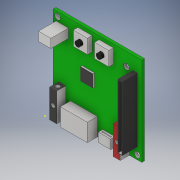
# Autodesk Inventor part: lab 04
Saved by Autodesk Inventor 2017 (Build 210142000, 142)
## iProperties
Created: 2016-10-26
Part Number: lab 04
Material: Generic
Document SubType Name: Modeling
Designer: radrajith
Density: 1 g/cm^3
Appearance: Default
Author: radrajith
Autodesk Inventor part; units mm, degrees
ref_plane "YZ Plane" through (0, 0, 0) normal (1, 0, 0) x (0, 1, 0)
ref_plane "XZ Plane" through (0, 0, 0) normal (0, 1, 0) x (-1, 0, 0)
ref_plane "XY Plane" through (0, 0, 0) normal (0, 0, 1) x (1, 0, 0)
sketch "Sketch1" plane through (0, 0, 0) normal (0, 0, 1) x (1, 0, 0)
  line L0 (0, 0) -> (50, 0)
  line L1 (50, 0) -> (50, 50)
  line L2 (50, 50) -> (0, 50)
  line L3 (0, 50) -> (0, 0)
  circle A0 centre (47.5, 2.5) radius 1.6
  circle A1 centre (41.39, 42.5) radius 1.6
  circle A2 centre (2.5, 47.5) radius 1.6
  dimension "d0" = 50
  dimension "d1" = 50
  dimension "d2" = 3.2
  dimension "d3" = 3.2
  dimension "d4" = 3.2
  constraints: 8 end point, 3 centre point, 2 parallel, 1 horizontal, 1 perpendicular
  measures "d0" distance of L2.end L1.end
  measures "d1" distance of L1.end L0.end
  measures "d2" diameter of A0
  measures "d3" diameter of A1
  measures "d4" diameter of A2
extrude "Extrusion1" add sketch "Sketch1" along normal blind 1.6
sketch "Sketch2" plane through (0, 0, 1.6) normal (0, 0, 1) x (1, 0, 0)
  line L0 (23.4, 30.52) -> (16.4, 30.52)
  line L1 (16.4, 30.52) -> (16.4, 23.52)
  line L2 (16.4, 23.52) -> (23.4, 23.52)
  line L3 (23.4, 23.52) -> (23.4, 30.52)
  point P0 (0, 0)
  dimension "d18" = 7
  dimension "d19" = 7
  constraints: 8 end point, 2 parallel, 1 horizontal, 1 perpendicular
  measures "d18" distance of L2.end L1.end
  measures "d19" distance of L1.end L0.end
extrude "Extrusion2" add sketch "Sketch2" along normal blind 1
sketch "Sketch3" plane through (0, 0, 1.6) normal (0, 0, 1) x (1, 0, 0)
  line L0 (47.541022, 6.34) -> (45.001022, 6.34)
  line L1 (45.001022, 6.34) -> (45.001022, 42.5)
  line L2 (45.001022, 42.5) -> (47.541022, 42.5)
  line L3 (47.541022, 42.5) -> (47.541022, 6.34)
  point P0 (0, 0)
  dimension "d11" = 2.54
  dimension "d12" = 36.16
  constraints: 8 end point, 2 parallel, 1 horizontal, 1 perpendicular
  measures "d11" distance of L1.end L2.end
  measures "d12" distance of L0.end L1.end
extrude "Extrusion3" add sketch "Sketch3" along normal blind 8.5
sketch "Sketch5" plane through (0, 0, 10.1) normal (0, 0, 1) x (1, 0, 0)
  line L0 (47.269103, 42.183511) -> (45.268765, 42.183511)
  line L1 (45.268765, 42.183511) -> (45.268765, 6.547483)
  line L2 (45.268765, 6.547483) -> (47.269103, 6.547483)
  line L3 (47.269103, 6.547483) -> (47.269103, 42.183511)
  point P0 (0, 0)
  constraints: 8 end point, 2 parallel, 1 horizontal, 1 perpendicular
extrude "Extrusion4" cut sketch "Sketch5" along normal mid plane 8
sketch "Sketch6" plane through (0, 0, 0) normal (0, -1, 0) x (1, 0, 0)
  line L0 (43, 1.6) -> (39, 1.6)
  line L1 (39, 1.6) -> (39, 6.75)
  line L2 (39, 6.75) -> (43, 6.75)
  line L3 (43, 6.75) -> (43, 1.6)
  line L4 (7.153325, 1.6) -> (3.153325, 1.6)
  line L5 (3.153325, 1.6) -> (3.153325, 6.75)
  line L6 (3.153325, 6.75) -> (7.153325, 6.75)
  line L7 (7.153325, 6.75) -> (7.153325, 1.6)
  line L8 (43, 1.6) -> (39, 1.6)
  line L9 (39, 1.6) -> (39, 6.75)
  line L10 (39, 6.75) -> (43, 6.75)
  line L11 (43, 6.75) -> (43, 1.6)
  point P0 (0, 0)
  dimension "d20" = 4
  dimension "d21" = 5.15
  dimension "d22" = 4
  dimension "d23" = 5.15
  dimension "d24" = 4
  dimension "d25" = 5.15
  constraints: 24 end point, 6 parallel, 3 horizontal, 3 perpendicular
  measures "d20" distance of L1.end L2.end
  measures "d21" distance of L0.end L1.end
  measures "d22" distance of L6.start L6.end
  measures "d23" distance of L5.start L6.start
  measures "d24" distance of L10.start L10.end
  measures "d25" distance of L9.start L10.start
extrude "Extrusion5" add sketch "Sketch6" against normal blind 16
hole "Hole1" at (41, 0, 4.175) direction (0, 1, 0) diameter 2.2 end through all
hole "Hole2" at (5.153325, 0, 4.175) direction (0, 1, 0) diameter 2.2 end through all
sketch "Sketch7" plane through (0, 0, 0) normal (0, -1, 0) x (1, 0, 0)
  line L0 (35, 4.100037) -> (28, 4.100037)
  line L1 (28, 4.100037) -> (28, 1.600037)
  line L2 (28, 1.600037) -> (35, 1.600037)
  line L3 (35, 1.600037) -> (35, 4.100037)
  point P0 (0, 0)
  dimension "d47" = 7
  dimension "d48" = 2.5
  constraints: 8 end point, 2 parallel, 1 horizontal, 1 perpendicular
  measures "d47" distance of L2.end L1.end
  measures "d48" distance of L1.end L0.end
extrude "Extrusion6" add sketch "Sketch7" against normal blind 5.1
shell "Shell1" thickness 1 removed faces 2 at (30.333333, 0, 3.266704) at (30.333333, 5.1, 3.266704)
sketch "Sketch8" plane through (0, 0, 0) normal (0, -1, 0) x (1, 0, 0)
  line L0 (25, 7.31808) -> (9.8, 7.31808)
  line L1 (9.8, 7.31808) -> (9.8, 1.59808)
  line L2 (9.8, 1.59808) -> (25, 1.59808)
  line L3 (25, 1.59808) -> (25, 7.31808)
  point P0 (0, 0)
  dimension "d52" = 15.2
  dimension "d56" = 5.72
  constraints: 8 end point, 2 parallel, 1 horizontal, 1 perpendicular
  measures "d52" distance of L2.end L1.end
  measures "d56" distance between parallel lines of L0 L2
extrude "Extrusion7" add sketch "Sketch8" against normal blind 10
sketch "Sketch10" plane through (0, 0, 0) normal (0, -1, 0) x (1, 0, 0)
  line L0 (11.3, 6.482537) -> (23.5, 6.482537)
  line L1 (23.5, 6.482537) -> (23.5, 2.838758)
  line L2 (23.5, 2.838758) -> (11.3, 2.838758)
  line L3 (11.3, 2.838758) -> (11.3, 6.482537)
  line L4 (9.8, 7.31808) -> (9.8, 1.6)
  line L5 (25, 7.31808) -> (25, 1.6)
  point P0 (0, 0)
  dimension "d57" = 1.5
  dimension "d58" = 1.5
  constraints: 8 end point, 2 parallel, 1 horizontal, 1 perpendicular
  measures "d57" distance between parallel lines of L3 L4
  measures "d58" distance between parallel lines of L5 L1
extrude "Extrusion8" cut sketch "Sketch10" against normal blind 8
sketch "Sketch11" plane through (0, 0, 1.6) normal (0, 0, 1) x (1, 0, 0)
  line L0 (22, 48) -> (14, 48)
  line L1 (14, 48) -> (14, 40)
  line L2 (14, 40) -> (22, 40)
  line L3 (22, 40) -> (22, 48)
  line L4 (26, 48) -> (34, 48)
  line L5 (34, 48) -> (34, 40)
  line L6 (34, 40) -> (26, 40)
  line L7 (26, 40) -> (26, 48)
  point P0 (0, 0)
  dimension "d61" = 8
  dimension "d62" = 8
  dimension "d63" = 8
  dimension "d64" = 8
  constraints: 16 end point, 4 parallel, 2 horizontal, 2 perpendicular, 1 point on line
  measures "d61" distance of L2.end L1.end
  measures "d62" distance of L1.end L0.end
  measures "d63" distance of L5.end L6.end
  measures "d64" distance of L4.end L5.end
extrude "Extrusion9" add sketch "Sketch11" along normal blind 2.6
sketch "Sketch16" plane through (0, 0, 4.2) normal (0, 0, 1) x (1, 0, 0)
  circle A0 centre (18, 44) radius 1.5
  circle A1 centre (30, 44) radius 1.5
  point P0 (0, 0)
  dimension "d69" = 3
  dimension "d70" = 3
  constraints: 2 centre point
  measures "d69" diameter of A0
  measures "d70" diameter of A1
extrude "Extrusion10" add sketch "Sketch16" along normal blind 1.7
sketch "Sketch17" plane through (0, 0, 1.6) normal (0, 0, 1) x (1, 0, 0)
  line L0 (1.7, 45) -> (8.7, 45)
  line L1 (8.7, 45) -> (8.7, 40)
  line L2 (8.7, 40) -> (1.7, 40)
  line L3 (1.7, 40) -> (1.7, 45)
  point P0 (0, 0)
  dimension "d73" = 7
  dimension "d74" = 5
  constraints: 8 end point, 2 parallel, 1 horizontal, 1 perpendicular
  measures "d73" distance of L1.end L2.end
  measures "d74" distance of L0.end L1.end
extrude "Extrusion11" add sketch "Sketch17" along normal blind 10
sketch "Sketch18" plane through (3.153325, 0, 6.75) normal (0, 0, 1) x (1, 0, 0)
  circle A0 centre (2, 8) radius 1.1
  circle A1 centre (37.952966, 8) radius 1.1
  point P0 (-3.153325, 0)
  dimension "d77" = 2.2
  dimension "d78" = 2.2
  constraints: 2 centre point
  measures "d77" diameter of A0
  measures "d78" diameter of A1
extrude "Extrusion12" cut sketch "Sketch18" against normal blind 4
sketch "Sketch19" plane through (0, 0, 1.6) normal (0, 0, 1) x (1, 0, 0)
  point P0 (0, 0)
sketch "Sketch20" plane through (0, 0, 6.1) normal (0, 0, 1) x (1, 0, 0)
  point P0 (0, 0)
body "Solid1"
